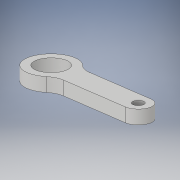
# Autodesk Inventor part: 小零件4
Saved by Autodesk Inventor 2017 (Build 210142000, 142)
## iProperties
Part Number: 小零件4
Material: 一般
Document SubType Name: Modeling
Designer: User
Density: 1 g/cm^3
Appearance: 預設
Author: User
Autodesk Inventor part; units mm, degrees
ref_plane "YZ Plane" through (0, 0, 0) normal (1, 0, 0) x (0, 1, 0)
ref_plane "XZ Plane" through (0, 0, 0) normal (0, 1, 0) x (-1, 0, 0)
ref_plane "XY Plane" through (0, 0, 0) normal (0, 0, 1) x (1, 0, 0)
sketch "草圖1" plane through (0, 0, 0) normal (0, 1, 0) x (-1, 0, 0)
  circle A0 centre (0, 0) radius 3.6
  arc A1 (-3.6485, -4.1822) -> (-3.6485, 4.1822) centre (0, 0) ccw
  line L0 (0, 0) -> (-23.9, 0)
  circle A2 centre (-23.9, 0) radius 2.95
  circle A3 centre (-23.9, 0) radius 1.25
  line L1 (-23.9, 2.95) -> (-6.9354, 2.95)
  line L2 (-23.9, -2.95) -> (-6.9354, -2.95)
  arc A4 (-6.9354, 2.95) -> (-3.6485, 4.1822) centre (-6.9354, 7.95) ccw
  arc A5 (-3.6485, -4.1822) -> (-6.9354, -2.95) centre (-6.9354, -7.95) ccw
  point P0 (-4.7011, 2.95)
  point P1 (-4.7011, -2.95)
  dimension "d0" = 7.2
  dimension "d1" = 11.1
  dimension "d2" = 23.9
  dimension "d3" = 5.9
  dimension "d4" = 2.5
  dimension "d5" = 5
  constraints: 10 point on circle, 6 centre point, 6 end point, 6 tangent, 4 coincident, 3 horizontal, 2 point on line, 1 equal radius
  measures "d0" diameter of A0
  measures "d1" diameter of A1
  measures "d2" distance of L0.start L0.end
  measures "d3" diameter of A2
  measures "d4" diameter of A3
  measures "d5" radius of A4
extrude "擠出1" add sketch "草圖1" along normal mid plane 3
